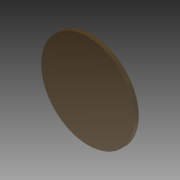
# Autodesk Inventor part: poly_filter
Saved by Autodesk Inventor 2015 (Build 190159000, 159)
## iProperties
Created: 2014-10-08
Part Number: poly_filter
Material: Polycarbonate, Smoke
Document SubType Name: Modeling
Designer: Adam
Density: 1.2 g/cm^3
Appearance: Polycarbonate - Smoked
Author: Adam
Autodesk Inventor part; units mm, degrees
ref_plane "YZ Plane" through (0, 0, 0) normal (1, 0, 0) x (0, 1, 0)
ref_plane "XZ Plane" through (0, 0, 0) normal (0, 1, 0) x (-1, 0, 0)
ref_plane "Work Plane1" through (0, 0, 0) normal (0, 0, 1) x (1, 0, 0)
sketch "Sketch1" plane through (0, 0, 0) normal (0, 0, 1) x (1, 0, 0)
  circle A0 centre (0, 0) radius 11 construction
  circle A1 centre (0, 0) radius 12.5
  circle A2 centre (0, 0) radius 13 construction
  point P0 (0, 0)
  dimension "d0" = 0.5
  constraints: 1 centre point, 1 coincident
  measures "d0" radial gap between concentric circles of A2 A1
extrude "Extrusion1" add sketch "Sketch1" along normal blind 1
body "Solid1"
